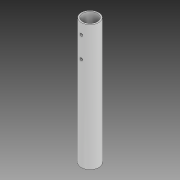
# Autodesk Inventor part: FE-110-004 Bottom Side Bar
Saved by Autodesk Inventor 2021 (Build 250183000, 183)
## iProperties
Created: 2021-01-11
Part Number: FE-110-004 Bottom Side Bar
Material: Aluminum 6061
Document SubType Name: Modeling
Density: 2.7 g/cm^3
Appearance: Aluminum - Dark
Autodesk Inventor part; units mm, degrees
ref_plane "YZ Plane" through (0, 0, 0) normal (1, 0, 0) x (0, 1, 0)
ref_plane "XZ Plane" through (0, 0, 0) normal (0, 1, 0) x (-1, 0, 0)
ref_plane "XY Plane" through (0, 0, 0) normal (0, 0, 1) x (1, 0, 0)
sketch "Sketch1" plane through (0, 0, 0) normal (0, 1, 0) x (-1, 0, 0)
  circle A0 centre (0, 0) radius 21.082
  circle A1 centre (0, 0) radius 17.526
  dimension "d0" = 42.164
  dimension "d1" = 35.052
  constraints: 2 centre point, 2 coincident
  measures "d0" diameter of A0
  measures "d1" diameter of A1
extrude "Extrusion1" add sketch "Sketch1" along normal mid plane 301.625
sketch "Sketch3" plane through (0, 0, 0) normal (0, 0, 1) x (1, 0, 0)
  circle A0 centre (0, 125.4125) radius 3.175
  circle A1 centre (0, 74.6125) radius 3.175
  line L0 (21.082, 150.8125) -> (-21.082, 150.8125) projected
  point P0 (0, 0)
  dimension "d10" = 25.4
  dimension "d11" = 76.2
  dimension "d12" = 6.35
  constraints: 2 centre point, 2 vertical alignment, 1 equal radius
  measures "d10" distance from line of A0.centre L0
  measures "d11" distance from line of A1.centre L0
  measures "d12" diameter of A0
extrude "Extrusion3" cut sketch "Sketch3" against normal through all both and the other way through all
body "Solid1"
